Autodesk Inventor part; units mm, degrees
(part 2 of 2)
sketch "Sketch120" plane through (0, 0, 52) normal (0, 0, -1) x (-1, 0, 0)
  line L0 (-5.5, 48.7965) -> (-5.5, 49.7965) projected
  line L1 (-5.5, 47.9965) -> (-5.5, 48.7965) projected
  line L2 (-5.5, 47.9965) -> (-5.5, 45.9965) projected
  line L3 (-5.5, 45.9965) -> (-5.5, 19.7965) projected
  line L4 (-5.5, 19.7965) -> (-5.5, 45.9965) projected
  line L5 (-5.5, 45.9965) -> (-5.5, 47.9965) projected
  line L6 (-5.5, 48.7965) -> (-5.5, 47.9965) projected
  line L7 (-5.5, 49.7965) -> (-5.5, 48.7965) projected
  line L8 (-5.5, -48.7965) -> (-5.5, -49.7965) projected
  line L9 (-5.5, -47.9965) -> (-5.5, -48.7965) projected
  line L10 (-5.5, -47.9965) -> (-5.5, -45.9965) projected
  line L11 (-5.5, -45.9965) -> (-5.5, -19.7965) projected
  line L12 (-5.5, -19.7965) -> (-5.5, -45.9965) projected
  line L13 (-5.5, -45.9965) -> (-5.5, -47.9965) projected
  line L14 (-5.5, -48.7965) -> (-5.5, -47.9965) projected
  line L15 (-5.5, -49.7965) -> (-5.5, -48.7965) projected
  line L16 (-6, 5.3855) -> (-6, 46.7965) projected
  line L17 (-6, -46.7965) -> (-6, -5.3855) projected
  line L18 (-6, 46.7965) -> (-3.5, 46.7965)
  line L19 (-3.5, 46.7965) -> (-3.5, 17.7965)
  line L20 (-3.5, 17.7965) -> (-6, 17.7965)
  line L21 (-6, 17.7965) -> (-6, 46.7965)
  line L22 (-6, -46.7965) -> (-3.5, -46.7965)
  line L23 (-3.5, -46.7965) -> (-3.5, -17.7965)
  line L24 (-3.5, -17.7965) -> (-6, -17.7965)
  line L25 (-6, -17.7965) -> (-6, -46.7965)
  point P0 (0, 0)
  dimension "d491" = 2
  dimension "d492" = 2
  dimension "d493" = 2
  constraints: 16 end point, 4 parallel, 2 horizontal, 2 perpendicular, 1 vertical alignment
  measures "d491" distance between parallel lines of L19 L3
  measures "d492" distance from line of L20 L3.end
  measures "d493" distance from line of L24 L11.end
extrude "Extrusion103" add sketch "Sketch120" along normal blind 2
sketch "Sketch123" plane through (9, -49.7965, 50) normal (1, 0, 0) x (0, 0, -1)
  line L0 (-2, 99.5929) -> (-5, 99.5929)
  line L1 (-5, 99.5929) -> (-5, 69.5929)
  line L2 (-5, 69.5929) -> (-2, 69.5929)
  line L3 (-2, 69.5929) -> (-2, 99.5929)
  line L4 (-3, 69.5929) -> (-32, 69.5929) projected
  line L5 (-3, 98.5929) -> (-3, 97.7929) projected
  line L6 (-3, 69.5929) -> (-35, 69.5929) projected
  line L7 (-19, 69.5929) -> (-19, 30)
  line L8 (-35, 30) -> (-3, 30) projected
  line L9 (0, 49.7965) -> (-70, 49.7965) projected
  line L10 (-2, 0) -> (-5, 0)
  line L11 (-5, 0) -> (-5, 30)
  line L12 (-5, 30) -> (-2, 30)
  line L13 (-2, 30) -> (-2, 0)
  line L14 (-36, 99.5929) -> (-33, 99.5929)
  line L15 (-33, 99.5929) -> (-33, 69.5929)
  line L16 (-33, 69.5929) -> (-36, 69.5929)
  line L17 (-36, 69.5929) -> (-36, 99.5929)
  line L18 (-33, 0) -> (-33, 30)
  line L19 (-36, 30) -> (-36, 0)
  line L20 (-33, 30) -> (-36, 30)
  line L21 (-36, 0) -> (-33, 0)
  point P0 (50, 49.7965)
  dimension "d494" = 2
  constraints: 34 end point, 12 symmetric about line, 2 midpoint, 2 parallel, 1 horizontal, 1 perpendicular, 1 point on line
  measures "d494" distance between parallel lines of L1 L5
extrude "Extrusion105" add sketch "Sketch123" against normal blind 1
sketch "Sketch125" plane through (5.5, -49.7965, 50) normal (1, 0, 0) x (0, 0, -1)
  line L0 (-36, 99.5929) -> (-2, 99.5929) projected
  line L1 (-35, 98.5929) -> (-36, 99.5929) projected
  line L2 (-35, 97.7929) -> (-35, 98.5929) projected
  line L3 (-35, 97.7929) -> (-35.6, 97.7929) projected
  line L4 (-35.6, 97.7929) -> (-35.6, 95.7929) projected
  line L5 (-35.6, 95.7929) -> (-35, 69.5929) projected
  line L6 (-3, 69.5929) -> (-35, 69.5929) projected
  line L7 (-3, 69.5929) -> (-2.4, 95.7929) projected
  line L8 (-2.4, 95.7929) -> (-2.4, 97.7929) projected
  line L9 (-2.4, 97.7929) -> (-3, 97.7929) projected
  line L10 (-3, 98.5929) -> (-3, 97.7929) projected
  line L11 (-2, 99.5929) -> (-3, 98.5929) projected
  line L12 (-2, 0) -> (-36, 0) projected
  line L13 (-3, 1) -> (-2, 0) projected
  line L14 (-3, 1.8) -> (-3, 1) projected
  line L15 (-3, 1.8) -> (-2.4, 1.8) projected
  line L16 (-2.4, 1.8) -> (-2.4, 3.8) projected
  line L17 (-2.4, 3.8) -> (-3, 30) projected
  line L18 (-35, 30) -> (-3, 30) projected
  line L19 (-35, 30) -> (-35.6, 3.8) projected
  line L20 (-35.6, 3.8) -> (-35.6, 1.8) projected
  line L21 (-35.6, 1.8) -> (-35, 1.8) projected
  line L22 (-35, 1) -> (-35, 1.8) projected
  line L23 (-36, 0) -> (-35, 1) projected
  point P0 (50, 49.7965)
extrude "Extrusion106" cut sketch "Sketch125" against normal blind 1
sketch "Sketch126" plane through (0, 0, 52) normal (0, 0, -1) x (-1, 0, 0)
  line L0 (21, 25.6491) -> (10, 19.2983)
  line L1 (10, 19.2983) -> (-1, 25.6491)
  line L2 (-1, 25.6491) -> (-1, 38.3509)
  line L3 (-1, 38.3509) -> (10, 44.7017)
  line L4 (10, 44.7017) -> (21, 38.3509)
  line L5 (21, 38.3509) -> (21, 25.6491)
  line L6 (0, 0) -> (77.78, 0) construction
  line L7 (21, -25.6491) -> (10, -19.2983)
  line L8 (10, -19.2983) -> (-1, -25.6491)
  line L9 (-1, -25.6491) -> (-1, -38.3509)
  line L10 (-1, -38.3509) -> (10, -44.7017)
  line L11 (10, -44.7017) -> (21, -38.3509)
  line L12 (21, -38.3509) -> (21, -25.6491)
  point P0 (10, 32)
  dimension "d499" = 32
  dimension "d500" = 22
  dimension "d501" = 10
  constraints: 26 end point, 6 symmetric about line, 1 horizontal, 1 vertical, 13 other
  measures "d499" vertical distance of L6.start point (10, 32)
  measures "d500" distance between parallel lines of L2 L5
  measures "d501" horizontal distance of L6.start point (10, 32)
extrude "Extrusion107" cut sketch "Sketch126" against normal through all
sketch "Sketch128" plane through (4.5, -49.7965, 50) normal (1, 0, 0) x (0, 0, -1)
  line L0 (-36, 99.5929) -> (-2, 99.5929) construction
  line L1 (-35, 98.5929) -> (-36, 99.5929) projected
  line L2 (-35, 97.7929) -> (-35, 98.5929) projected
  line L3 (-35.6, 97.7929) -> (-35, 97.7929) projected
  line L4 (-35.6, 95.7929) -> (-35.6, 97.7929) projected
  line L5 (-35, 69.5929) -> (-35.6, 95.7929) projected
  line L6 (-3, 69.5929) -> (-35, 69.5929) projected
  line L7 (-2.4, 95.7929) -> (-3, 69.5929) projected
  line L8 (-2.4, 97.7929) -> (-2.4, 95.7929) projected
  line L9 (-3, 97.7929) -> (-2.4, 97.7929) projected
  line L10 (-3, 98.5929) -> (-3, 97.7929) projected
  line L11 (-2, 99.5929) -> (-3, 98.5929) projected
  line L12 (-2.4, 97.7929) -> (-2.4, 99.1929)
  line L13 (-2.4, 99.1929) -> (-3, 98.5929)
  line L14 (-3, 98.5929) -> (-3, 97.7929)
  line L15 (-2.4, 97.7929) -> (-3, 97.7929)
  line L16 (-35.6, 97.7929) -> (-35.6, 99.1929)
  line L17 (-35.6, 99.1929) -> (-35, 98.5929)
  line L18 (-35, 97.7929) -> (-35, 98.5929)
  line L19 (-35, 97.7929) -> (-35.6, 97.7929)
  point P0 (50, 49.7965)
  constraints: 16 end point, 5 collinear, 2 point on line, 1 parallel, 1 perpendicular, 1 vertical
extrude "Extrusion108" cut sketch "Sketch128" along normal blind 3.5
sketch "Sketch129" plane through (4.5, -49.7965, 50) normal (1, 0, 0) x (0, 0, -1)
  line L0 (-36, 99.5929) -> (-2, 99.5929) projected
  line L1 (-35.6, 99.1929) -> (-36, 99.5929) projected
  line L2 (-35.6, 99.1929) -> (-35.6, 95.7929) projected
  line L3 (-35, 69.5929) -> (-35.6, 95.7929) projected
  line L4 (-3, 69.5929) -> (-35, 69.5929) construction
  line L5 (-2.4, 95.7929) -> (-3, 69.5929) projected
  line L6 (-2.4, 99.1929) -> (-2.4, 95.7929) projected
  line L7 (-2, 99.5929) -> (-2.4, 99.1929) projected
  line L8 (-35, 69.5929) -> (-35, 99.5929)
  line L9 (-35, 99.5929) -> (-3, 99.5929)
  line L10 (-3, 99.5929) -> (-3, 69.5929)
  line L11 (-35, 98.5929) -> (-33.2, 98.5929)
  line L12 (-33.2, 98.5929) -> (-33.2, 96.5929)
  line L13 (-33.2, 96.5929) -> (-35, 96.5929)
  line L14 (-35, 96.5929) -> (-35, 98.5929)
  line L15 (-35, 98.5929) -> (-35.6, 98.5929)
  line L16 (-35, 96.5929) -> (-35.6, 96.5929)
  line L17 (-35.6, 96.5929) -> (-35.6, 98.5929)
  point P0 (50, 49.7965)
  dimension "d506" = 1.8
  dimension "d507" = 27
  dimension "d508" = 2
  constraints: 20 end point, 4 perpendicular, 4 point on line, 3 parallel, 2 horizontal, 1 collinear
  measures "d506" distance of L12.end L13.end
  measures "d507" distance between parallel lines of L4 L13
  measures "d508" distance of L11.end L12.end
extrude "Extrusion109" add sketch "Sketch129" along normal blind 3.5 contours L11 L12 L13 L8 | L8 L16 L2 L15
mirror "Mirror1" about plane through (0, 0, 0) normal (0, 1, 0) of "Extrusion108", "Extrusion109"
sketch "Sketch130" plane through (57.5, 0, 120) normal (0.8660254, -0.5, 0) x (0, 0, -1)
  line L0 (35, -10) -> (5, -10)
  line L1 (5, -10) -> (5, -12)
  line L2 (5, -12) -> (35, -12)
  line L3 (35, -12) -> (35, -10)
  line L4 (40, 0) -> (0, 0) projected
  line L5 (35, -15) -> (5, -15)
  line L6 (5, -15) -> (5, -17)
  line L7 (5, -17) -> (35, -17)
  line L8 (35, -17) -> (35, -15)
  line L9 (35, -15) -> (5, -15)
  line L10 (5, -15) -> (5, -17)
  line L11 (5, -17) -> (35, -17)
  line L12 (35, -17) -> (35, -15)
  line L13 (35, -20) -> (5, -20)
  line L14 (5, -20) -> (5, -22)
  line L15 (5, -22) -> (35, -22)
  line L16 (35, -22) -> (35, -20)
  line L17 (35, -25) -> (5, -25)
  line L18 (5, -25) -> (5, -27)
  line L19 (5, -27) -> (35, -27)
  line L20 (35, -27) -> (35, -25)
  point P0 (120, -28.75)
  point P1 (20, -10)
  point P2 (20, 0)
  point P3 (20, -15)
  point P4 (20, -15)
  point P5 (20, -20)
  point P6 (20, -25)
  dimension "d511" = 30
  dimension "d512" = 2
  dimension "d513" = 10
  dimension "d516" = 5
  dimension "d525" = 5
  constraints: 40 end point, 2 midpoint, 2 parallel, 2 vertical, 1 collinear, 1 horizontal, 1 perpendicular, 1 vertical alignment, 35 other
  measures "d511" distance of L1.end L2.end
  measures "d512" distance of L0.end L1.end
  measures "d513" distance between parallel lines of L4 L0
  measures "d516" distance of L0.start L5.start
  measures "d525" distance of L0.start L9.start
extrude "Extrusion110" cut sketch "Sketch130" against normal blind 15
body "Solid2"
